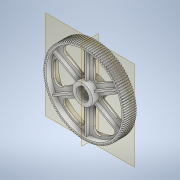
# Autodesk Inventor part: 正齿轮2
Saved by Autodesk Inventor 2020 (Build 240168000, 168)
## iProperties
CustomPartVersion: 1
Created: 2021-06-09
Part Number: 正齿轮2
Material: Steel
Document SubType Name: Modeling
Designer: dell
Categories: <?xml version="1.0" encoding="UTF-16"?> <MemberInstance><Categories><FamilyTemplate><FamilyTemplateParameter ValueType="xs:double" Id="1" ObjectReferenceKey="da_z" ObjectType="kUserParameterObject"/><FamilyTemplateParameter ValueType="xs:double" Id="2" ObjectReferenceKey="da_b" ObjectType="kUserParameterObject"/><FamilyTemplateParameter ValueType="xs:double" Id="3" ObjectReferenceKey="da_beta" ObjectType="kUserParameterObject"/><FamilyTemplateParameter ValueType="xs:double" Id="4" ObjectReferenceKey="da_da" ObjectType="kUserParameterObject"/><FamilyTemplateParameter ValueType="xs:double" Id="5" ObjectReferenceKey="da_aw" ObjectType="kUserParameterObject"/><FamilyTemplateParameter ValueType="xs:string" Id="6" ObjectReferenceKey="EAIAABAAAACIAQAAAAAAAIAAAAAAAAAA" ObjectType="83910656" SubObjectId="SurfaceGeometry"/></FamilyTemplate><ParamToTemplateMap><ParamToTemplate CategoryParameter="//CategoryParameter[@InternalName='046C89C9-8512-4d59-83FE-43B91F4F132A']" TemplateParameter="1"/><ParamToTemplate CategoryParameter="//CategoryParameter[@InternalName='2552DF32-E462-4b46-AEBF-C6C7768E72AC']" TemplateParameter="2"/><ParamToTemplate CategoryParameter="//CategoryParameter[@InternalName='C9EE641D-15FC-4fae-A226-E94C4372FDD7']" TemplateParameter="3"/><ParamToTemplate><ParamToTemplate CategoryParameter="//CategoryParameter[@InternalName='00B6519A-459B-49c7-AD84-2E56D39A5744']" ConstantValue="0.000000"/></ParamToTemplate><ParamToTemplate><ParamToTemplate CategoryParameter="//CategoryParameter[@InternalName='04B31F0E-C7A6-4894-AA32-9629BEFACF47']" ConstantValue="1.000000"/></ParamToTemplate><ParamToTemplate><ParamToTemplate CategoryParameter="//CategoryParameter[@InternalName='43CBEC2E-7847-49e7-A936-2F7889FCB2D9']" ConstantValue="0.250000"/></ParamToTemplate><ParamToTemplate><ParamToTemplate CategoryParameter="//CategoryParameter[@InternalName='B1EFC894-105D-4ebd-86BF-FA20ED196853']" ConstantValue="0.350000"/></ParamToTemplate><ParamToTemplate><ParamToTemplate CategoryParameter="//CategoryParameter[@InternalName='51175063-3D10-4879-93E8-6246FE8B403D']" ConstantValue="2060000000.000000"/></ParamToTemplate><ParamToTemplate><ParamToTemplate CategoryParameter="//CategoryParameter[@InternalName='A3A52E27-4454-46a9-B0BD-C932399B70AF']" ConstantValue="0.300000"/></ParamToTemplate><ParamToTemplate><ParamToTemplate CategoryParameter="//CategoryParameter[@InternalName='91B76062-C214-41d9-B1B9-14D2AB99603D']" ConstantValue="0.400000"/></ParamToTemplate><ParamToTemplate><ParamToTemplate CategoryParameter="//CategoryParameter[@InternalName='374E806E-8B8A-4dda-A9AA-1039D6500AD2']" ConstantValue="2.500000"/></ParamToTemplate><ParamToTemplate><ParamToTemplate CategoryParameter="//CategoryParameter[@InternalName='2D373A89-B862-43d6-8D0B-0CBF12AB9F6C']" ConstantValue="0.349066"/></ParamToTemplate><ParamToTemplate CategoryParameter="//CategoryParameter[@InternalName='37777632-D6A2-4fac-9D53-DB8ACD95C989']" TemplateParameter="4"/><ParamToTemplate CategoryParameter="//CategoryParameter[@InternalName='FD1017F1-B727-4f7e-9707-0F86F1FF9423']" TemplateParameter="5"/><ParamToTemplate><ParamToTemplate CategoryParameter="//CategoryParameter[@InternalName='9E1B4470-B2D3-4ff1-B813-535BB4CDF51A']" ConstantValue="3960000.000000"/></ParamToTemplate><ParamToTemplate><ParamToTemplate CategoryParameter="//CategoryParameter[@InternalName='F8452263-BFF6-458c-9FB1-07C4B99E95CD']" ConstantValue="4800000.000000"/></ParamToTemplate><ParamToTemplate><ParamToTemplate CategoryParameter="//CategoryParameter[@InternalName='3E3BB259-FD49-497f-8171-6EBC954A3479']" ConstantValue="0.000000"/></ParamToTemplate><ParamToTemplate CategoryParameter="//CategoryParameter[@InternalName='27C3BAF2-7550-4e4b-AE2C-0DB134B7D9B7']" TemplateParameter="6"/></ParamToTemplateMap><Category DisplayName="Gear" InternalName="DC85795E-93AB-48d5-8EEE-5A27447B64BD" Mnemonic="Gear"><CategoryParameter DisplayName="z" InternalName="046C89C9-8512-4d59-83FE-43B91F4F132A" Mnemonic="z"/><CategoryParameter DisplayName="b" InternalName="2552DF32-E462-4b46-AEBF-C6C7768E72AC" Mnemonic="b"/><CategoryParameter DisplayName="||b|" InternalName="C9EE641D-15FC-4fae-A226-E94C4372FDD7" Mnemonic="beta"/><CategoryParameter DisplayName="x" InternalName="00B6519A-459B-49c7-AD84-2E56D39A5744" Mnemonic="x"/><CategoryParameter DisplayName="a*" InternalName="04B31F0E-C7A6-4894-AA32-9629BEFACF47" Mnemonic="a"/><CategoryParameter DisplayName="c*" InternalName="43CBEC2E-7847-49e7-A936-2F7889FCB2D9" Mnemonic="c"/><CategoryParameter DisplayName="r|.f|*" InternalName="B1EFC894-105D-4ebd-86BF-FA20ED196853" Mnemonic="rf"/><CategoryParameter DisplayName="E" InternalName="51175063-3D10-4879-93E8-6246FE8B403D" Mnemonic="E"/><CategoryParameter DisplayName="||m|" InternalName="A3A52E27-4454-46a9-B0BD-C932399B70AF" Mnemonic="mi"/><Category DisplayName="SpurGear" InternalName="26C5A22E-A91E-4dfd-A3B3-23CCAFAE1764" Mnemonic="SpurGear"><CategoryParameter DisplayName="m" InternalName="91B76062-C214-41d9-B1B9-14D2AB99603D" Mnemonic="m"/><CategoryParameter DisplayName="P" InternalName="374E806E-8B8A-4dda-A9AA-1039D6500AD2" Mnemonic="PP"/><CategoryParameter DisplayName="||a|" InternalName="2D373A89-B862-43d6-8D0B-0CBF12AB9F6C" Mnemonic="alpha"/><CategoryParameter DisplayName="d|.a|" InternalName="37777632-D6A2-4fac-9D53-DB8ACD95C989" Mnemonic="da"/><CategoryParameter DisplayName="a|.w|" InternalName="FD1017F1-B727-4f7e-9707-0F86F1FF9423" Mnemonic="aw"/><CategoryParameter DisplayName="||s||.Flim|" InternalName="9E1B4470-B2D3-4ff1-B813-535BB4CDF51A" Mnemonic="sFlim"/><CategoryParameter DisplayName="||s||.Hlim|" InternalName="F8452263-BFF6-458c-9FB1-07C4B99E95CD" Mnemonic="sHlim"/><CategoryParameter DisplayName="类型" InternalName="3E3BB259-FD49-497f-8171-6EBC954A3479" Mnemonic="type"/><CategoryParameter DisplayName="PitchDiameter" InternalName="27C3BAF2-7550-4e4b-AE2C-0DB134B7D9B7" Mnemonic="IDS_PITCHDIAM"/></Category></Category></Categories></MemberInstance>
Density: 1 g/cm^3
Appearance: Steel
Author: dell
Autodesk Inventor part; units mm, degrees
(part 1 of 2)
sketch "Sketch1" plane through (0, 0, 0) normal (0, 0, 1) x (1, 0, 0)
  circle A0 centre (0, 0) radius 242
  dimension "d0" = 484
  constraints: 1 centre point
  measures "d0" diameter of A0
extrude "Extrusion1" add sketch "Sketch1" along normal blind 73
ref_plane "Work Plane2" through (0, 0, 36.5) normal (0, 0, 1) x (1, 0, 0)
sketch "Sketch2" plane through (0, 0, 0) normal (0, 0, -1) x (-1, 0, 0)
  circle A0 centre (0, 0) radius 242 projected
  circle A1 centre (0, 0) radius 238
  dimension "d3" = 476
  constraints: 1 centre point, 1 coincident
  measures "d3" diameter of A1
surface extrude "中径" sketch "Sketch2" against normal through all shown no curves A1
ref_plane "Work Plane8" through (0, 0, 0) normal (0.9996515, 0.0263969, 0) x (0, 0, 1)
ref_plane "Work Plane9" through (0, 0, 0) normal (1, 0, 0) x (0, 1, 0)
spur gear teeth "正齿轮" teeth 119 pitch diameter 476 tip diameter 484 root diameter 466 face width 73 start plane through (0, 0, 0) normal (0, 0, -1) x (-1, 0, 0)
sketch "草图3" plane through (0, 0, 73) normal (0, 0, 1) x (1, 0, 0)
  circle A0 centre (0, 0) radius 37.5
  circle A1 centre (0, 0) radius 60
  line L0 (43.1421, 10) -> (31.1421, 10)
  line L1 (31.1421, 10) -> (31.1421, -10)
  line L2 (31.1421, -10) -> (43.1421, -10)
  line L3 (43.1421, -10) -> (43.1421, 10)
  line L4 (-338.7926, 0) -> (338.7926, 0) construction
  arc A2 (-14.3663, 241.5732) -> (-16.9009, 232.3862) centre (40.0791, 221.6091) ccw projected
  arc A3 (-16.9009, 232.3862) -> (-19.9668, 232.1429) centre (0, 0) ccw projected
  arc A4 (-19.9668, 232.1429) -> (-23.9188, 240.8151) centre (-74.5336, 212.5128) ccw projected
  arc A5 (-23.9188, 240.8151) -> (-27.0954, 240.4784) centre (0, 0) ccw projected
  arc A6 (-27.0954, 240.4784) -> (-29.1416, 231.1704) centre (28.3278, 223.4155) ccw projected
  arc A7 (-29.1416, 231.1704) -> (-32.1904, 230.7656) centre (0, 0) ccw projected
  arc A8 (-32.1904, 230.7656) -> (-36.5946, 239.2171) centre (-85.6452, 208.2831) ccw projected
  arc A9 (-36.5946, 239.2171) -> (-39.749, 238.7133) centre (0, 0) ccw projected
  arc A10 (-39.749, 238.7133) -> (-41.3011, 229.3103) centre (16.4975, 224.5992) ccw projected
  arc A11 (-41.3011, 229.3103) -> (-44.3243, 228.7452) centre (0, 0) ccw projected
  arc A12 (-44.3243, 228.7452) -> (-49.1684, 236.9525) centre (-96.518, 203.4729) ccw projected
  arc A13 (-49.1684, 236.9525) -> (-52.2918, 236.2828) centre (0, 0) ccw projected
  arc A14 (-52.2918, 236.2828) -> (-53.3455, 226.8111) centre (4.6212, 225.1568) ccw projected
  arc A15 (-53.3455, 226.8111) -> (-56.3346, 226.0872) centre (0, 0) ccw projected
  arc A16 (-56.3346, 226.0872) -> (-61.6051, 234.0274) centre (-107.1219, 198.0956) ccw projected
  arc A17 (-61.6051, 234.0274) -> (-64.6888, 233.1938) centre (0, 0) ccw projected
  arc A18 (-64.6888, 233.1938) -> (-65.2412, 223.6797) centre (-7.268, 225.0869) ccw projected
  arc A19 (-65.2412, 223.6797) -> (-68.188, 222.799) centre (0, 0) ccw projected
  arc A20 (-68.188, 222.799) -> (-73.8701, 230.45) centre (-117.4271, 192.1661) ccw projected
  arc A21 (-73.8701, 230.45) -> (-76.9055, 229.4549) centre (0, 0) ccw projected
  arc A22 (-76.9055, 229.4549) -> (-76.955, 219.9248) centre (-19.1369, 224.3897) ccw projected
  arc A23 (-76.955, 219.9248) -> (-79.8512, 218.8899) centre (0, 0) ccw projected
  arc A24 (-79.8512, 218.8899) -> (-85.9292, 226.2303) centre (-127.4051, 185.701) ccw projected
  arc A25 (-85.9292, 226.2303) -> (-88.9079, 225.0764) centre (0, 0) ccw projected
  arc A26 (-88.9079, 225.0764) -> (-88.4544, 215.557) centre (-30.9525, 223.067) ccw projected
  arc A27 (-88.4544, 215.557) -> (-91.2919, 214.3707) centre (0, 0) ccw projected
  arc A28 (-91.2919, 214.3707) -> (-97.7489, 221.3801) centre (-137.028, 178.7184) ccw projected
  arc A29 (-97.7489, 221.3801) -> (-100.6625, 220.0706) centre (0, 0) ccw projected
  arc A30 (-100.6625, 220.0706) -> (-99.7072, 210.5884) centre (-42.6818, 221.1226) ccw projected
  arc A31 (-99.7072, 210.5884) -> (-102.4782, 209.254) centre (0, 0) ccw projected
  arc A32 (-102.4782, 209.254) -> (-109.2961, 215.9129) centre (-146.269, 171.2376) ccw projected
  arc A33 (-109.2961, 215.9129) -> (-112.1365, 214.4514) centre (0, 0) ccw projected
  arc A34 (-112.1365, 214.4514) -> (-110.6821, 205.0328) centre (-54.2921, 218.5619) ccw projected
  arc A35 (-110.6821, 205.0328) -> (-113.3788, 203.554) centre (0, 0) ccw projected
  arc A36 (-113.3788, 203.554) -> (-120.5386, 209.8438) centre (-155.1023, 163.2796) ccw projected
  arc A37 (-120.5386, 209.8438) -> (-123.298, 208.2345) centre (0, 0) ccw projected
  arc A38 (-123.298, 208.2345) -> (-121.3486, 198.9058) centre (-65.7511, 215.3921) ccw projected
  arc A39 (-121.3486, 198.9058) -> (-123.9635, 197.2867) centre (0, 0) ccw projected
  arc A40 (-123.9635, 197.2867) -> (-131.4452, 203.1899) centre (-163.5033, 154.8665) ccw projected
  arc A41 (-131.4452, 203.1899) -> (-134.1158, 201.4372) centre (0, 0) ccw projected
  arc A42 (-134.1158, 201.4372) -> (-131.6768, 192.2244) centre (-77.0269, 211.6218) ccw projected
  arc A43 (-131.6768, 192.2244) -> (-134.2026, 190.4696) centre (0, 0) ccw projected
  arc A44 (-134.2026, 190.4696) -> (-141.9855, 195.9697) centre (-171.4485, 146.0217) ccw projected
  arc A45 (-141.9855, 195.9697) -> (-144.5598, 194.0785) centre (0, 0) ccw projected
  arc A46 (-144.5598, 194.0785) -> (-141.638, 185.0072) centre (-88.088, 207.2618) ccw projected
  arc A47 (-141.638, 185.0072) -> (-144.0677, 183.1216) centre (0, 0) ccw projected
  arc A48 (-144.0677, 183.1216) -> (-152.13, 188.2033) centre (-178.916, 136.77) ccw projected
  arc A49 (-152.13, 188.2033) -> (-154.6009, 186.1788) centre (0, 0) ccw projected
  arc A50 (-154.6009, 186.1788) -> (-151.2044, 177.2744) centre (-98.9035, 202.3241) ccw projected
  arc A51 (-151.2044, 177.2744) -> (-153.5312, 175.2631) centre (0, 0) ccw projected
  arc A52 (-153.5312, 175.2631) -> (-161.8505, 179.9123) centre (-185.8847, 127.137) ccw projected
  arc A53 (-161.8505, 179.9123) -> (-164.2111, 177.7602) centre (0, 0) ccw projected
  arc A54 (-164.2111, 177.7602) -> (-160.3494, 169.0475) centre (-109.4434, 196.8225) ccw projected
  arc A55 (-160.3494, 169.0475) -> (-162.5668, 166.9162) centre (0, 0) ccw projected
  arc A56 (-162.5668, 166.9162) -> (-171.1198, 171.1198) centre (-192.3354, 117.1497) ccw projected
  arc A57 (-171.1198, 171.1198) -> (-173.3636, 168.8462) centre (0, 0) ccw projected
  arc A58 (-173.3636, 168.8462) -> (-169.0475, 160.3494) centre (-119.6783, 190.7723) ccw projected
  arc A59 (-169.0475, 160.3494) -> (-171.1493, 158.1041) centre (0, 0) ccw projected
  arc A60 (-171.1493, 158.1041) -> (-179.9123, 161.8505) centre (-198.2499, 106.8359) ccw projected
  arc A61 (-179.9123, 161.8505) -> (-182.033, 159.4616) centre (0, 0) ccw projected
  arc A62 (-182.033, 159.4616) -> (-177.2744, 151.2044) centre (-129.5796, 184.1904) ccw projected
  arc A63 (-177.2744, 151.2044) -> (-179.2548, 148.8513) centre (0, 0) ccw projected
  arc A64 (-179.2548, 148.8513) -> (-188.2033, 152.13) centre (-203.612, 96.2243) ccw projected
  arc A65 (-188.2033, 152.13) -> (-190.1949, 149.6325) centre (0, 0) ccw projected
  arc A66 (-190.1949, 149.6325) -> (-185.0072, 141.638) centre (-139.1197, 177.0951) ccw projected
  arc A67 (-185.0072, 141.638) -> (-186.8607, 139.1836) centre (0, 0) ccw projected
  arc A68 (-186.8607, 139.1836) -> (-195.9697, 141.9855) centre (-208.4065, 85.3445) ccw projected
  arc A69 (-195.9697, 141.9855) -> (-197.8268, 139.3864) centre (0, 0) ccw projected
  arc A70 (-197.8268, 139.3864) -> (-192.2244, 131.6768) centre (-148.2721, 169.5062) ccw projected
  arc A71 (-192.2244, 131.6768) -> (-193.9457, 129.128) centre (0, 0) ccw projected
  arc A72 (-193.9457, 129.128) -> (-203.1899, 131.4452) centre (-212.6201, 74.2269) ccw projected
  arc A73 (-203.1899, 131.4452) -> (-204.9073, 128.7518) centre (0, 0) ccw projected
  arc A74 (-204.9073, 128.7518) -> (-198.9058, 121.3486) centre (-157.0112, 161.4448) ccw projected
  arc A75 (-198.9058, 121.3486) -> (-200.4902, 118.7125) centre (0, 0) ccw projected
  arc A76 (-200.4902, 118.7125) -> (-209.8438, 120.5386) centre (-216.2412, 62.9023) ccw projected
  arc A77 (-209.8438, 120.5386) -> (-211.4166, 117.7583) centre (0, 0) ccw projected
  arc A78 (-211.4166, 117.7583) -> (-205.0328, 110.6821) centre (-165.3127, 152.9335) ccw projected
  arc A79 (-205.0328, 110.6821) -> (-206.4759, 107.9661) centre (0, 0) ccw projected
  arc A80 (-206.4759, 107.9661) -> (-215.9129, 109.2961) centre (-219.2595, 51.4024) ccw projected
  arc A81 (-215.9129, 109.2961) -> (-217.3367, 106.4366) centre (0, 0) ccw projected
  arc A82 (-217.3367, 106.4366) -> (-210.5884, 99.7072) centre (-173.1534, 143.996) ccw projected
  arc A83 (-210.5884, 99.7072) -> (-211.8861, 96.9188) centre (0, 0) ccw projected
  arc A84 (-211.8861, 96.9188) -> (-221.3801, 97.7489) centre (-221.6667, 39.7593) ccw projected
  arc A85 (-221.3801, 97.7489) -> (-222.6511, 94.8182) centre (0, 0) ccw projected
  arc A86 (-222.6511, 94.8182) -> (-215.557, 88.4544) centre (-180.5115, 134.6571) ccw projected
  arc A87 (-215.557, 88.4544) -> (-216.7058, 85.6014) centre (0, 0) ccw projected
  arc A88 (-216.7058, 85.6014) -> (-226.2303, 85.9292) centre (-223.4561, 28.0054) ccw projected
  arc A89 (-226.2303, 85.9292) -> (-227.3449, 82.9356) centre (0, 0) ccw projected
  arc A90 (-227.3449, 82.9356) -> (-219.9248, 76.955) centre (-187.3666, 124.9429) ccw projected
  arc A91 (-219.9248, 76.955) -> (-220.9214, 74.0454) centre (0, 0) ccw projected
  arc A92 (-220.9214, 74.0454) -> (-230.45, 73.8701) centre (-224.6227, 16.1734) ccw projected
  arc A93 (-230.45, 73.8701) -> (-231.405, 70.8218) centre (0, 0) ccw projected
  arc A94 (-231.405, 70.8218) -> (-223.6797, 65.2412) centre (-193.6994, 114.8804) ccw projected
  arc A95 (-223.6797, 65.2412) -> (-224.5213, 62.283) centre (0, 0) ccw projected
  arc A96 (-224.5213, 62.283) -> (-234.0274, 61.6051) centre (-225.1632, 4.2963) ccw projected
  arc A97 (-234.0274, 61.6051) -> (-234.8201, 58.5107) centre (0, 0) ccw projected
  arc A98 (-234.8201, 58.5107) -> (-226.8111, 53.3455) centre (-199.4923, 104.4978) ccw projected
  arc A99 (-226.8111, 53.3455) -> (-227.4954, 50.347) centre (0, 0) ccw projected
  arc A100 (-227.4954, 50.347) -> (-236.9525, 49.1684) centre (-225.0762, -7.5928) ccw projected
  arc A101 (-236.9525, 49.1684) -> (-237.5808, 46.0364) centre (0, 0) ccw projected
  arc A102 (-237.5808, 46.0364) -> (-229.3103, 41.3011) centre (-204.7292, 93.8239) ccw projected
  arc A103 (-229.3103, 41.3011) -> (-229.8355, 38.2707) centre (0, 0) ccw projected
  arc A104 (-229.8355, 38.2707) -> (-239.2171, 36.5946) centre (-224.3618, -19.4607) ccw projected
  arc A105 (-239.2171, 36.5946) -> (-239.6793, 33.4338) centre (0, 0) ccw projected
  arc A106 (-239.6793, 33.4338) -> (-231.1704, 29.1416) centre (-209.3954, 82.8884) ccw projected
  arc A107 (-231.1704, 29.1416) -> (-231.5349, 26.0877) centre (0, 0) ccw projected
  arc A108 (-231.5349, 26.0877) -> (-240.8151, 23.9188) centre (-223.0221, -31.2743) ccw projected
  arc A109 (-240.8151, 23.9188) -> (-241.1098, 20.7381) centre (0, 0) ccw projected
  arc A110 (-241.1098, 20.7381) -> (-232.3862, 16.9009) centre (-213.4781, 71.722) ccw projected
  arc A111 (-232.3862, 16.9009) -> (-232.5891, 13.832) centre (0, 0) ccw projected
  arc A112 (-232.5891, 13.832) -> (-241.7418, 11.1764) centre (-221.0608, -43.0008) ccw projected
  arc A113 (-241.7418, 11.1764) -> (-241.8682, 7.9845) centre (0, 0) ccw projected
  arc A114 (-241.8682, 7.9845) -> (-232.9543, 4.6131) centre (-216.9658, 60.3557) ccw projected
  arc A115 (-232.9543, 4.6131) -> (-232.9949, 1.5378) centre (0, 0) ccw projected
  arc A116 (-232.9949, 1.5378) -> (-241.9947, -1.5972) centre (-218.4833, -54.6074) ccw projected
  arc A117 (-241.9947, -1.5972) -> (-241.9526, -4.7913) centre (0, 0) ccw projected
  arc A118 (-241.9526, -4.7913) -> (-232.8731, -7.6876) centre (-219.8487, 48.8211) ccw projected
  arc A119 (-232.8731, -7.6876) -> (-232.7514, -10.7607) centre (0, 0) ccw projected
  arc A120 (-232.7514, -10.7607) -> (-241.5732, -14.3663) centre (-215.2969, -66.0619) ccw projected
  arc A121 (-241.5732, -14.3663) -> (-241.3625, -17.5537) centre (0, 0) ccw projected
  arc A122 (-241.3625, -17.5537) -> (-232.1429, -19.9668) centre (-222.1189, 37.1505) ccw projected
  arc A123 (-232.1429, -19.9668) -> (-231.8591, -23.0293) centre (0, 0) ccw projected
  arc A124 (-231.8591, -23.0293) -> (-240.4784, -27.0954) centre (-211.5105, -77.3322) ccw projected
  arc A125 (-240.4784, -27.0954) -> (-240.0998, -30.2673) centre (0, 0) ccw projected
  arc A126 (-240.0998, -30.2673) -> (-230.7656, -32.1904) centre (-223.7699, 25.3763) ccw projected
  arc A127 (-230.7656, -32.1904) -> (-230.3206, -35.2336) centre (0, 0) ccw projected
  arc A128 (-230.3206, -35.2336) -> (-238.7133, -39.749) centre (-207.1345, -88.387) ccw projected
  arc A129 (-238.7133, -39.749) -> (-238.1678, -42.8964) centre (0, 0) ccw projected
  arc A130 (-238.1678, -42.8964) -> (-228.7452, -44.3243) centre (-224.7973, 13.5314) ccw projected
  arc A131 (-228.7452, -44.3243) -> (-228.1402, -47.3398) centre (0, 0) ccw projected
  arc A132 (-228.1402, -47.3398) -> (-236.2828, -52.2918) centre (-202.1812, -99.1954) ccw projected
  arc A133 (-236.2828, -52.2918) -> (-235.572, -55.406) centre (0, 0) ccw projected
  arc A134 (-235.572, -55.406) -> (-226.0872, -56.3346) centre (-225.1982, 1.6488) ccw projected
  arc A135 (-226.0872, -56.3346) -> (-225.3239, -59.314) centre (0, 0) ccw projected
  arc A136 (-225.3239, -59.314) -> (-233.1938, -64.6888) centre (-196.6643, -109.7273) ccw projected
  arc A137 (-233.1938, -64.6888) -> (-232.3196, -67.7612) centre (0, 0) ccw projected
  arc A138 (-232.3196, -67.7612) -> (-222.799, -68.188) centre (-224.9714, -10.2384) ccw projected
  arc A139 (-222.799, -68.188) -> (-221.8796, -71.1229) centre (0, 0) ccw projected
  arc A140 (-221.8796, -71.1229) -> (-229.4549, -76.9055) centre (-190.5994, -119.9534) ccw projected
  arc A141 (-229.4549, -76.9055) -> (-228.4198, -79.9275) centre (0, 0) ccw projected
  arc A142 (-228.4198, -79.9275) -> (-218.8899, -79.8512) centre (-224.1175, -22.0971) ccw projected
  arc A143 (-218.8899, -79.8512) -> (-217.8168, -82.7335) centre (0, 0) ccw projected
  arc A144 (-217.8168, -82.7335) -> (-225.0764, -88.9079) centre (-184.0032, -129.8452) ccw projected
  arc A145 (-225.0764, -88.9079) -> (-223.8832, -91.8711) centre (0, 0) ccw projected
  arc A146 (-223.8832, -91.8711) -> (-214.3707, -91.2919) centre (-222.639, -33.8942) ccw projected
  arc A147 (-214.3707, -91.2919) -> (-213.147, -94.1136) centre (0, 0) ccw projected
  arc A148 (-213.147, -94.1136) -> (-220.0706, -100.6625) centre (-176.8941, -139.3751) ccw projected
  arc A149 (-220.0706, -100.6625) -> (-218.7227, -103.5586) centre (0, 0) ccw projected
  arc A150 (-218.7227, -103.5586) -> (-209.254, -102.4782) centre (-220.54, -45.5968) ccw projected
  arc A151 (-209.254, -102.4782) -> (-207.8831, -105.2313) centre (0, 0) ccw projected
  arc A152 (-207.8831, -105.2313) -> (-214.4514, -112.1365) centre (-169.292, -148.5165) ccw projected
  arc A153 (-214.4514, -112.1365) -> (-212.9526, -114.9574) centre (0, 0) ccw projected
  arc A154 (-212.9526, -114.9574) -> (-203.554, -113.3788) centre (-217.8262, -57.1723) ccw projected
  arc A155 (-203.554, -113.3788) -> (-202.0397, -116.0558) centre (0, 0) ccw projected
  arc A156 (-202.0397, -116.0558) -> (-208.2345, -123.298) centre (-161.2181, -157.244) ccw projected
  arc A157 (-208.2345, -123.298) -> (-206.5889, -126.0359) centre (0, 0) ccw projected
  arc A158 (-206.5889, -126.0359) -> (-197.2867, -123.9635) centre (-214.5054, -68.5885) ccw projected
  arc A159 (-197.2867, -123.9635) -> (-195.6333, -126.5568) centre (0, 0) ccw projected
  arc A160 (-195.6333, -126.5568) -> (-201.4372, -134.1158) centre (-152.6948, -165.5332) ccw projected
  arc A161 (-201.4372, -134.1158) -> (-199.6494, -136.763) centre (0, 0) ccw projected
  arc A162 (-199.6494, -136.763) -> (-190.4696, -134.2026) centre (-210.5867, -79.8135) ccw projected
  arc A163 (-190.4696, -134.2026) -> (-188.6816, -136.705) centre (0, 0) ccw projected
  arc A164 (-188.6816, -136.705) -> (-194.0785, -144.5598) centre (-143.746, -173.361) ccw projected
  arc A165 (-194.0785, -144.5598) -> (-192.1534, -147.109) centre (0, 0) ccw projected
  arc A166 (-192.1534, -147.109) -> (-183.1216, -144.0677) centre (-206.081, -90.8161) ccw projected
  arc A167 (-183.1216, -144.0677) -> (-181.204, -146.4722) centre (0, 0) ccw projected
  arc A168 (-181.204, -146.4722) -> (-186.1788, -154.6009) centre (-134.3964, -180.7057) ccw projected
  arc A169 (-186.1788, -154.6009) -> (-184.1219, -157.0449) centre (0, 0) ccw projected
  arc A170 (-184.1219, -157.0449) -> (-175.2631, -153.5312) centre (-201.001, -101.5655) ccw projected
  arc A171 (-175.2631, -153.5312) -> (-173.2213, -155.8312) centre (0, 0) ccw projected
  arc A172 (-173.2213, -155.8312) -> (-177.7602, -164.2111) centre (-124.6724, -187.5467) ccw projected
  arc A173 (-177.7602, -164.2111) -> (-175.5772, -166.5432) centre (0, 0) ccw projected
  arc A174 (-175.5772, -166.5432) -> (-166.9162, -162.5668) centre (-195.3607, -112.0318) ccw projected
  arc A175 (-166.9162, -162.5668) -> (-164.7559, -164.7559) centre (0, 0) ccw projected
  arc A176 (-164.7559, -164.7559) -> (-168.8462, -173.3636) centre (-114.6008, -193.8649) ccw projected
  arc A177 (-168.8462, -173.3636) -> (-166.5432, -175.5772) centre (0, 0) ccw projected
  arc A178 (-166.5432, -175.5772) -> (-158.1041, -171.1493) centre (-189.1759, -122.186) ccw projected
  arc A179 (-158.1041, -171.1493) -> (-155.8312, -173.2213) centre (0, 0) ccw projected
  arc A180 (-155.8312, -173.2213) -> (-159.4616, -182.033) centre (-104.2098, -199.6429) ccw projected
  arc A181 (-159.4616, -182.033) -> (-157.0449, -184.1219) centre (0, 0) ccw projected
  arc A182 (-157.0449, -184.1219) -> (-148.8513, -179.2548) centre (-182.4639, -131.9995) ccw projected
  arc A183 (-148.8513, -179.2548) -> (-146.4722, -181.204) centre (0, 0) ccw projected
  arc A184 (-146.4722, -181.204) -> (-149.6325, -190.1949) centre (-93.5283, -204.8643) ccw projected
  arc A185 (-149.6325, -190.1949) -> (-147.109, -192.1534) centre (0, 0) ccw projected
  arc A186 (-147.109, -192.1534) -> (-139.1836, -186.8607) centre (-175.2433, -141.4451) ccw projected
  arc A187 (-139.1836, -186.8607) -> (-136.705, -188.6816) centre (0, 0) ccw projected
  arc A188 (-136.705, -188.6816) -> (-139.3864, -197.8268) centre (-82.5862, -209.5148) ccw projected
  arc A189 (-139.3864, -197.8268) -> (-136.763, -199.6494) centre (0, 0) ccw projected
  arc A190 (-136.763, -199.6494) -> (-129.128, -193.9457) centre (-167.5343, -150.4966) ccw projected
  arc A191 (-129.128, -193.9457) -> (-126.5568, -195.6333) centre (0, 0) ccw projected
  arc A192 (-126.5568, -195.6333) -> (-128.7518, -204.9073) centre (-71.4139, -213.5814) ccw projected
  arc A193 (-128.7518, -204.9073) -> (-126.0359, -206.5889) centre (0, 0) ccw projected
  arc A194 (-126.0359, -206.5889) -> (-118.7125, -200.4902) centre (-159.3583, -159.1285) ccw projected
  arc A195 (-118.7125, -200.4902) -> (-116.0558, -202.0397) centre (0, 0) ccw projected
  arc A196 (-116.0558, -202.0397) -> (-117.7583, -211.4166) centre (-60.0425, -217.0526) ccw projected
  arc A197 (-117.7583, -211.4166) -> (-114.9574, -212.9526) centre (0, 0) ccw projected
  arc A198 (-114.9574, -212.9526) -> (-107.9661, -206.4759) centre (-150.7382, -167.3169) ccw projected
  arc A199 (-107.9661, -206.4759) -> (-105.2313, -207.8831) centre (0, 0) ccw projected
  arc A200 (-105.2313, -207.8831) -> (-106.4366, -217.3367) centre (-48.5038, -219.9189) ccw projected
  arc A201 (-106.4366, -217.3367) -> (-103.5586, -218.7227) centre (0, 0) ccw projected
  arc A202 (-103.5586, -218.7227) -> (-96.9188, -211.8861) centre (-141.6979, -175.039) ccw projected
  arc A203 (-96.9188, -211.8861) -> (-94.1136, -213.147) centre (0, 0) ccw projected
  arc A204 (-94.1136, -213.147) -> (-94.8182, -222.6511) centre (-36.8299, -222.1722) ccw projected
  arc A205 (-94.8182, -222.6511) -> (-91.8711, -223.8832) centre (0, 0) ccw projected
  arc A206 (-91.8711, -223.8832) -> (-85.6014, -216.7058) centre (-132.2627, -182.2732) ccw projected
  arc A207 (-85.6014, -216.7058) -> (-82.7335, -217.8168) centre (0, 0) ccw projected
  arc A208 (-82.7335, -217.8168) -> (-82.9356, -227.3449) centre (-25.0534, -223.8063) ccw projected
  arc A209 (-82.9356, -227.3449) -> (-79.9275, -228.4198) centre (0, 0) ccw projected
  arc A210 (-79.9275, -228.4198) -> (-74.0454, -220.9214) centre (-122.4588, -188.9994) ccw projected
  arc A211 (-74.0454, -220.9214) -> (-71.1229, -221.8796) centre (0, 0) ccw projected
  arc A212 (-71.1229, -221.8796) -> (-70.8218, -231.405) centre (-13.207, -224.8166) ccw projected
  arc A213 (-70.8218, -231.405) -> (-67.7612, -232.3196) centre (0, 0) ccw projected
  arc A214 (-67.7612, -232.3196) -> (-62.283, -224.5213) centre (-112.3136, -195.1989) ccw projected
  arc A215 (-62.283, -224.5213) -> (-59.314, -225.3239) centre (0, 0) ccw projected
  arc A216 (-59.314, -225.3239) -> (-58.5107, -234.8201) centre (-1.3238, -225.2003) ccw projected
  arc A217 (-58.5107, -234.8201) -> (-55.406, -235.572) centre (0, 0) ccw projected
  arc A218 (-55.406, -235.572) -> (-50.347, -227.4954) centre (-101.8554, -200.8542) ccw projected
  arc A219 (-50.347, -227.4954) -> (-47.3398, -228.1402) centre (0, 0) ccw projected
  arc A220 (-47.3398, -228.1402) -> (-46.0364, -237.5808) centre (10.563, -224.9564) ccw projected
  arc A221 (-46.0364, -237.5808) -> (-42.8964, -238.1678) centre (0, 0) ccw projected
  arc A222 (-42.8964, -238.1678) -> (-38.2707, -229.8355) centre (-91.1133, -205.9498) ccw projected
  arc A223 (-38.2707, -229.8355) -> (-35.2336, -230.3206) centre (0, 0) ccw projected
  arc A224 (-35.2336, -230.3206) -> (-33.4338, -239.6793) centre (22.4205, -224.0854) ccw projected
  arc A225 (-33.4338, -239.6793) -> (-30.2673, -240.0998) centre (0, 0) ccw projected
  arc A226 (-30.2673, -240.0998) -> (-26.0877, -231.5349) centre (-80.1173, -210.4713) ccw projected
  arc A227 (-26.0877, -231.5349) -> (-23.0293, -231.8591) centre (0, 0) ccw projected
  arc A228 (-23.0293, -231.8591) -> (-20.7381, -241.1098) centre (34.2154, -222.5899) ccw projected
  arc A229 (-20.7381, -241.1098) -> (-17.5537, -241.3625) centre (0, 0) ccw projected
  arc A230 (-17.5537, -241.3625) -> (-13.832, -232.5891) centre (-68.8979, -214.4062) ccw projected
  arc A231 (-13.832, -232.5891) -> (-10.7607, -232.7514) centre (0, 0) ccw projected
  arc A232 (-10.7607, -232.7514) -> (-7.9845, -241.8682) centre (45.915, -220.4739) ccw projected
  arc A233 (-7.9845, -241.8682) -> (-4.7913, -241.9526) centre (0, 0) ccw projected
  arc A234 (-4.7913, -241.9526) -> (-1.5378, -232.9949) centre (-57.4866, -217.7435) ccw projected
  arc A235 (-1.5378, -232.9949) -> (1.5378, -232.9949) centre (0, 0) ccw projected
  arc A236 (1.5378, -232.9949) -> (4.7913, -241.9526) centre (57.4866, -217.7435) ccw projected
  arc A237 (4.7913, -241.9526) -> (7.9845, -241.8682) centre (0, 0) ccw projected
  arc A238 (7.9845, -241.8682) -> (10.7607, -232.7514) centre (-45.915, -220.4739) ccw projected
  arc A239 (10.7607, -232.7514) -> (13.832, -232.5891) centre (0, 0) ccw projected
  arc A240 (13.832, -232.5891) -> (17.5537, -241.3625) centre (68.8979, -214.4062) ccw projected
  arc A241 (17.5537, -241.3625) -> (20.7381, -241.1098) centre (0, 0) ccw projected
  arc A242 (20.7381, -241.1098) -> (23.0293, -231.8591) centre (-34.2154, -222.5899) ccw projected
  arc A243 (23.0293, -231.8591) -> (26.0877, -231.5349) centre (0, 0) ccw projected
  arc A244 (26.0877, -231.5349) -> (30.2673, -240.0998) centre (80.1173, -210.4713) ccw projected
  arc A245 (30.2673, -240.0998) -> (33.4338, -239.6793) centre (0, 0) ccw projected
  arc A246 (33.4338, -239.6793) -> (35.2336, -230.3206) centre (-22.4205, -224.0854) ccw projected
  arc A247 (35.2336, -230.3206) -> (38.2707, -229.8355) centre (0, 0) ccw projected
  arc A248 (38.2707, -229.8355) -> (42.8964, -238.1678) centre (91.1133, -205.9498) ccw projected
  arc A249 (42.8964, -238.1678) -> (46.0364, -237.5808) centre (0, 0) ccw projected
  arc A250 (46.0364, -237.5808) -> (47.3398, -228.1402) centre (-10.563, -224.9564) ccw projected
  arc A251 (47.3398, -228.1402) -> (50.347, -227.4954) centre (0, 0) ccw projected
  arc A252 (50.347, -227.4954) -> (55.406, -235.572) centre (101.8554, -200.8542) ccw projected
  arc A253 (55.406, -235.572) -> (58.5107, -234.8201) centre (0, 0) ccw projected
  arc A254 (58.5107, -234.8201) -> (59.314, -225.3239) centre (1.3238, -225.2003) ccw projected
  arc A255 (59.314, -225.3239) -> (62.283, -224.5213) centre (0, 0) ccw projected
  arc A256 (62.283, -224.5213) -> (67.7612, -232.3196) centre (112.3136, -195.1989) ccw projected
  arc A257 (67.7612, -232.3196) -> (70.8218, -231.405) centre (0, 0) ccw projected
  arc A258 (70.8218, -231.405) -> (71.1229, -221.8796) centre (13.207, -224.8166) ccw projected
  arc A259 (71.1229, -221.8796) -> (74.0454, -220.9214) centre (0, 0) ccw projected
  arc A260 (74.0454, -220.9214) -> (79.9275, -228.4198) centre (122.4588, -188.9994) ccw projected
  arc A261 (79.9275, -228.4198) -> (82.9356, -227.3449) centre (0, 0) ccw projected
  arc A262 (82.9356, -227.3449) -> (82.7335, -217.8168) centre (25.0534, -223.8063) ccw projected
  arc A263 (82.7335, -217.8168) -> (85.6014, -216.7058) centre (0, 0) ccw projected
  arc A264 (85.6014, -216.7058) -> (91.8711, -223.8832) centre (132.2627, -182.2732) ccw projected
  arc A265 (91.8711, -223.8832) -> (94.8182, -222.6511) centre (0, 0) ccw projected
  arc A266 (94.8182, -222.6511) -> (94.1136, -213.147) centre (36.8299, -222.1722) ccw projected
  arc A267 (94.1136, -213.147) -> (96.9188, -211.8861) centre (0, 0) ccw projected
  arc A268 (96.9188, -211.8861) -> (103.5586, -218.7227) centre (141.6979, -175.039) ccw projected
  arc A269 (103.5586, -218.7227) -> (106.4366, -217.3367) centre (0, 0) ccw projected
  arc A270 (106.4366, -217.3367) -> (105.2313, -207.8831) centre (48.5038, -219.9189) ccw projected
  arc A271 (105.2313, -207.8831) -> (107.9661, -206.4759) centre (0, 0) ccw projected
  arc A272 (107.9661, -206.4759) -> (114.9574, -212.9526) centre (150.7382, -167.3169) ccw projected
  arc A273 (114.9574, -212.9526) -> (117.7583, -211.4166) centre (0, 0) ccw projected
  arc A274 (117.7583, -211.4166) -> (116.0558, -202.0397) centre (60.0425, -217.0526) ccw projected
  arc A275 (116.0558, -202.0397) -> (118.7125, -200.4902) centre (0, 0) ccw projected
  arc A276 (118.7125, -200.4902) -> (126.0359, -206.5889) centre (159.3583, -159.1285) ccw projected
  arc A277 (126.0359, -206.5889) -> (128.7518, -204.9073) centre (0, 0) ccw projected
  arc A278 (128.7518, -204.9073) -> (126.5568, -195.6333) centre (71.4139, -213.5814) ccw projected
  arc A279 (126.5568, -195.6333) -> (129.128, -193.9457) centre (0, 0) ccw projected
  arc A280 (129.128, -193.9457) -> (136.763, -199.6494) centre (167.5343, -150.4966) ccw projected
  arc A281 (136.763, -199.6494) -> (139.3864, -197.8268) centre (0, 0) ccw projected
  arc A282 (139.3864, -197.8268) -> (136.705, -188.6816) centre (82.5862, -209.5148) ccw projected
  arc A283 (136.705, -188.6816) -> (139.1836, -186.8607) centre (0, 0) ccw projected
  arc A284 (139.1836, -186.8607) -> (147.109, -192.1534) centre (175.2433, -141.4451) ccw projected
  arc A285 (147.109, -192.1534) -> (149.6325, -190.1949) centre (0, 0) ccw projected
  arc A286 (149.6325, -190.1949) -> (146.4722, -181.204) centre (93.5283, -204.8643) ccw projected
  arc A287 (146.4722, -181.204) -> (148.8513, -179.2548) centre (0, 0) ccw projected
  arc A288 (148.8513, -179.2548) -> (157.0449, -184.1219) centre (182.4639, -131.9995) ccw projected
  arc A289 (157.0449, -184.1219) -> (159.4616, -182.033) centre (0, 0) ccw projected
  arc A290 (159.4616, -182.033) -> (155.8312, -173.2213) centre (104.2098, -199.6429) ccw projected
  arc A291 (155.8312, -173.2213) -> (158.1041, -171.1493) centre (0, 0) ccw projected
  arc A292 (158.1041, -171.1493) -> (166.5432, -175.5772) centre (189.1759, -122.186) ccw projected
  arc A293 (166.5432, -175.5772) -> (168.8462, -173.3636) centre (0, 0) ccw projected
  arc A294 (168.8462, -173.3636) -> (164.7559, -164.7559) centre (114.6008, -193.8649) ccw projected
  arc A295 (164.7559, -164.7559) -> (166.9162, -162.5668) centre (0, 0) ccw projected
  arc A296 (166.9162, -162.5668) -> (175.5772, -166.5432) centre (195.3607, -112.0318) ccw projected
  arc A297 (175.5772, -166.5432) -> (177.7602, -164.2111) centre (0, 0) ccw projected
  arc A298 (177.7602, -164.2111) -> (173.2213, -155.8312) centre (124.6724, -187.5467) ccw projected
  arc A299 (173.2213, -155.8312) -> (175.2631, -153.5312) centre (0, 0) ccw projected
  arc A300 (175.2631, -153.5312) -> (184.1219, -157.0449) centre (201.001, -101.5655) ccw projected
  arc A301 (184.1219, -157.0449) -> (186.1788, -154.6009) centre (0, 0) ccw projected
  arc A302 (186.1788, -154.6009) -> (181.204, -146.4722) centre (134.3964, -180.7057) ccw projected
  arc A303 (181.204, -146.4722) -> (183.1216, -144.0677) centre (0, 0) ccw projected
  arc A304 (183.1216, -144.0677) -> (192.1534, -147.109) centre (206.081, -90.8161) ccw projected
  arc A305 (192.1534, -147.109) -> (194.0785, -144.5598) centre (0, 0) ccw projected
  arc A306 (194.0785, -144.5598) -> (188.6816, -136.705) centre (143.746, -173.361) ccw projected
  arc A307 (188.6816, -136.705) -> (190.4696, -134.2026) centre (0, 0) ccw projected
  arc A308 (190.4696, -134.2026) -> (199.6494, -136.763) centre (210.5867, -79.8135) ccw projected
  arc A309 (199.6494, -136.763) -> (201.4372, -134.1158) centre (0, 0) ccw projected
  arc A310 (201.4372, -134.1158) -> (195.6333, -126.5568) centre (152.6948, -165.5332) ccw projected
  arc A311 (195.6333, -126.5568) -> (197.2867, -123.9635) centre (0, 0) ccw projected
  arc A312 (197.2867, -123.9635) -> (206.5889, -126.0359) centre (214.5054, -68.5885) ccw projected
  arc A313 (206.5889, -126.0359) -> (208.2345, -123.298) centre (0, 0) ccw projected
  arc A314 (208.2345, -123.298) -> (202.0397, -116.0558) centre (161.2181, -157.244) ccw projected
  arc A315 (202.0397, -116.0558) -> (203.554, -113.3788) centre (0, 0) ccw projected
  arc A316 (203.554, -113.3788) -> (212.9526, -114.9574) centre (217.8262, -57.1723) ccw projected
  arc A317 (212.9526, -114.9574) -> (214.4514, -112.1365) centre (0, 0) ccw projected
  arc A318 (214.4514, -112.1365) -> (207.8831, -105.2313) centre (169.292, -148.5165) ccw projected
  arc A319 (207.8831, -105.2313) -> (209.254, -102.4782) centre (0, 0) ccw projected
  arc A320 (209.254, -102.4782) -> (218.7227, -103.5586) centre (220.54, -45.5968) ccw projected
  arc A321 (218.7227, -103.5586) -> (220.0706, -100.6625) centre (0, 0) ccw projected
  arc A322 (220.0706, -100.6625) -> (213.147, -94.1136) centre (176.8941, -139.3751) ccw projected
  arc A323 (213.147, -94.1136) -> (214.3707, -91.2919) centre (0, 0) ccw projected
  arc A324 (214.3707, -91.2919) -> (223.8832, -91.8711) centre (222.639, -33.8942) ccw projected
  arc A325 (223.8832, -91.8711) -> (225.0764, -88.9079) centre (0, 0) ccw projected
  arc A326 (225.0764, -88.9079) -> (217.8168, -82.7335) centre (184.0032, -129.8452) ccw projected
  arc A327 (217.8168, -82.7335) -> (218.8899, -79.8512) centre (0, 0) ccw projected
  arc A328 (218.8899, -79.8512) -> (228.4198, -79.9275) centre (224.1175, -22.0971) ccw projected
  arc A329 (228.4198, -79.9275) -> (229.4549, -76.9055) centre (0, 0) ccw projected
  arc A330 (229.4549, -76.9055) -> (221.8796, -71.1229) centre (190.5994, -119.9534) ccw projected
  arc A331 (221.8796, -71.1229) -> (222.799, -68.188) centre (0, 0) ccw projected
  arc A332 (222.799, -68.188) -> (232.3196, -67.7612) centre (224.9714, -10.2384) ccw projected
  arc A333 (232.3196, -67.7612) -> (233.1938, -64.6888) centre (0, 0) ccw projected
  arc A334 (233.1938, -64.6888) -> (225.3239, -59.314) centre (196.6643, -109.7273) ccw projected
  arc A335 (225.3239, -59.314) -> (226.0872, -56.3346) centre (0, 0) ccw projected
  arc A336 (226.0872, -56.3346) -> (235.572, -55.406) centre (225.1982, 1.6488) ccw projected
  arc A337 (235.572, -55.406) -> (236.2828, -52.2918) centre (0, 0) ccw projected
  arc A338 (236.2828, -52.2918) -> (228.1402, -47.3398) centre (202.1812, -99.1954) ccw projected
  arc A339 (228.1402, -47.3398) -> (228.7452, -44.3243) centre (0, 0) ccw projected
  arc A340 (228.7452, -44.3243) -> (238.1678, -42.8964) centre (224.7973, 13.5314) ccw projected
  arc A341 (238.1678, -42.8964) -> (238.7133, -39.749) centre (0, 0) ccw projected
  arc A342 (238.7133, -39.749) -> (230.3206, -35.2336) centre (207.1345, -88.387) ccw projected
  arc A343 (230.3206, -35.2336) -> (230.7656, -32.1904) centre (0, 0) ccw projected
  arc A344 (230.7656, -32.1904) -> (240.0998, -30.2673) centre (223.7699, 25.3763) ccw projected
  arc A345 (240.0998, -30.2673) -> (240.4784, -27.0954) centre (0, 0) ccw projected
  arc A346 (240.4784, -27.0954) -> (231.8591, -23.0293) centre (211.5105, -77.3322) ccw projected
  arc A347 (231.8591, -23.0293) -> (232.1429, -19.9668) centre (0, 0) ccw projected
  arc A348 (232.1429, -19.9668) -> (241.3625, -17.5537) centre (222.1189, 37.1505) ccw projected
  arc A349 (241.3625, -17.5537) -> (241.5732, -14.3663) centre (0, 0) ccw projected
  arc A350 (241.5732, -14.3663) -> (232.7514, -10.7607) centre (215.2969, -66.0619) ccw projected
  arc A351 (232.7514, -10.7607) -> (232.8731, -7.6876) centre (0, 0) ccw projected
  arc A352 (232.8731, -7.6876) -> (241.9526, -4.7913) centre (219.8487, 48.8211) ccw projected
  arc A353 (241.9526, -4.7913) -> (241.9947, -1.5972) centre (0, 0) ccw projected
  arc A354 (241.9947, -1.5972) -> (232.9949, 1.5378) centre (218.4833, -54.6074) ccw projected
  arc A355 (232.9949, 1.5378) -> (232.9543, 4.6131) centre (0, 0) ccw projected
  arc A356 (232.9543, 4.6131) -> (241.8682, 7.9845) centre (216.9658, 60.3557) ccw projected
  arc A357 (241.8682, 7.9845) -> (241.7418, 11.1764) centre (0, 0) ccw projected
  arc A358 (241.7418, 11.1764) -> (232.5891, 13.832) centre (221.0608, -43.0008) ccw projected
  arc A359 (232.5891, 13.832) -> (232.3862, 16.9009) centre (0, 0) ccw projected
  arc A360 (232.3862, 16.9009) -> (241.1098, 20.7381) centre (213.4781, 71.722) ccw projected
  arc A361 (241.1098, 20.7381) -> (240.8151, 23.9188) centre (0, 0) ccw projected
  arc A362 (240.8151, 23.9188) -> (231.5349, 26.0877) centre (223.0221, -31.2743) ccw projected
  arc A363 (231.5349, 26.0877) -> (231.1704, 29.1416) centre (0, 0) ccw projected
  arc A364 (231.1704, 29.1416) -> (239.6793, 33.4338) centre (209.3954, 82.8884) ccw projected
  arc A365 (239.6793, 33.4338) -> (239.2171, 36.5946) centre (0, 0) ccw projected
  arc A366 (239.2171, 36.5946) -> (229.8355, 38.2707) centre (224.3618, -19.4607) ccw projected
  arc A367 (229.8355, 38.2707) -> (229.3103, 41.3011) centre (0, 0) ccw projected
  arc A368 (229.3103, 41.3011) -> (237.5808, 46.0364) centre (204.7292, 93.8239) ccw projected
  arc A369 (237.5808, 46.0364) -> (236.9525, 49.1684) centre (0, 0) ccw projected
  arc A370 (236.9525, 49.1684) -> (227.4954, 50.347) centre (225.0762, -7.5928) ccw projected
  arc A371 (227.4954, 50.347) -> (226.8111, 53.3455) centre (0, 0) ccw projected
  arc A372 (226.8111, 53.3455) -> (234.8201, 58.5107) centre (199.4923, 104.4978) ccw projected
  arc A373 (234.8201, 58.5107) -> (234.0274, 61.6051) centre (0, 0) ccw projected
  arc A374 (234.0274, 61.6051) -> (224.5213, 62.283) centre (225.1632, 4.2963) ccw projected
  arc A375 (224.5213, 62.283) -> (223.6797, 65.2412) centre (0, 0) ccw projected
  arc A376 (223.6797, 65.2412) -> (231.405, 70.8218) centre (193.6994, 114.8804) ccw projected
  arc A377 (231.405, 70.8218) -> (230.45, 73.8701) centre (0, 0) ccw projected
  arc A378 (230.45, 73.8701) -> (220.9214, 74.0454) centre (224.6227, 16.1734) ccw projected
  arc A379 (220.9214, 74.0454) -> (219.9248, 76.955) centre (0, 0) ccw projected
  arc A380 (219.9248, 76.955) -> (227.3449, 82.9356) centre (187.3666, 124.9429) ccw projected
  arc A381 (227.3449, 82.9356) -> (226.2303, 85.9292) centre (0, 0) ccw projected
  arc A382 (226.2303, 85.9292) -> (216.7058, 85.6014) centre (223.4561, 28.0054) ccw projected
  arc A383 (216.7058, 85.6014) -> (215.557, 88.4544) centre (0, 0) ccw projected
  arc A384 (215.557, 88.4544) -> (222.6511, 94.8182) centre (180.5115, 134.6571) ccw projected
  arc A385 (222.6511, 94.8182) -> (221.3801, 97.7489) centre (0, 0) ccw projected
  arc A386 (221.3801, 97.7489) -> (211.8861, 96.9188) centre (221.6667, 39.7593) ccw projected
  arc A387 (211.8861, 96.9188) -> (210.5884, 99.7072) centre (0, 0) ccw projected
  arc A388 (210.5884, 99.7072) -> (217.3367, 106.4366) centre (173.1534, 143.996) ccw projected
  arc A389 (217.3367, 106.4366) -> (215.9129, 109.2961) centre (0, 0) ccw projected
  arc A390 (215.9129, 109.2961) -> (206.4759, 107.9661) centre (219.2595, 51.4024) ccw projected
  arc A391 (206.4759, 107.9661) -> (205.0328, 110.6821) centre (0, 0) ccw projected
  arc A392 (205.0328, 110.6821) -> (211.4166, 117.7583) centre (165.3127, 152.9335) ccw projected
  arc A393 (211.4166, 117.7583) -> (209.8438, 120.5386) centre (0, 0) ccw projected
  arc A394 (209.8438, 120.5386) -> (200.4902, 118.7125) centre (216.2412, 62.9023) ccw projected
  arc A395 (200.4902, 118.7125) -> (198.9058, 121.3486) centre (0, 0) ccw projected
  arc A396 (198.9058, 121.3486) -> (204.9073, 128.7518) centre (157.0112, 161.4448) ccw projected
  arc A397 (204.9073, 128.7518) -> (203.1899, 131.4452) centre (0, 0) ccw projected
  arc A398 (203.1899, 131.4452) -> (193.9457, 129.128) centre (212.6201, 74.2269) ccw projected
  arc A399 (193.9457, 129.128) -> (192.2244, 131.6768) centre (0, 0) ccw projected
  arc A400 (192.2244, 131.6768) -> (197.8268, 139.3864) centre (148.2721, 169.5062) ccw projected
  arc A401 (197.8268, 139.3864) -> (195.9697, 141.9855) centre (0, 0) ccw projected
  arc A402 (195.9697, 141.9855) -> (186.8607, 139.1836) centre (208.4065, 85.3445) ccw projected
  arc A403 (186.8607, 139.1836) -> (185.0072, 141.638) centre (0, 0) ccw projected
  arc A404 (185.0072, 141.638) -> (190.1949, 149.6325) centre (139.1197, 177.0951) ccw projected
  arc A405 (190.1949, 149.6325) -> (188.2033, 152.13) centre (0, 0) ccw projected
  arc A406 (188.2033, 152.13) -> (179.2548, 148.8513) centre (203.612, 96.2243) ccw projected
  arc A407 (179.2548, 148.8513) -> (177.2744, 151.2044) centre (0, 0) ccw projected
  arc A408 (177.2744, 151.2044) -> (182.033, 159.4616) centre (129.5796, 184.1904) ccw projected
  arc A409 (182.033, 159.4616) -> (179.9123, 161.8505) centre (0, 0) ccw projected
  arc A410 (179.9123, 161.8505) -> (171.1493, 158.1041) centre (198.2499, 106.8359) ccw projected
  arc A411 (171.1493, 158.1041) -> (169.0475, 160.3494) centre (0, 0) ccw projected
  arc A412 (169.0475, 160.3494) -> (173.3636, 168.8462) centre (119.6783, 190.7723) ccw projected
  arc A413 (173.3636, 168.8462) -> (171.1198, 171.1198) centre (0, 0) ccw projected
  arc A414 (171.1198, 171.1198) -> (162.5668, 166.9162) centre (192.3354, 117.1497) ccw projected
  arc A415 (162.5668, 166.9162) -> (160.3494, 169.0475) centre (0, 0) ccw projected
  arc A416 (160.3494, 169.0475) -> (164.2111, 177.7602) centre (109.4434, 196.8225) ccw projected
  arc A417 (164.2111, 177.7602) -> (161.8505, 179.9123) centre (0, 0) ccw projected
  arc A418 (161.8505, 179.9123) -> (153.5312, 175.2631) centre (185.8847, 127.137) ccw projected
  arc A419 (153.5312, 175.2631) -> (151.2044, 177.2744) centre (0, 0) ccw projected
  arc A420 (151.2044, 177.2744) -> (154.6009, 186.1788) centre (98.9035, 202.3241) ccw projected
  arc A421 (154.6009, 186.1788) -> (152.13, 188.2033) centre (0, 0) ccw projected
  arc A422 (152.13, 188.2033) -> (144.0677, 183.1216) centre (178.916, 136.77) ccw projected
  arc A423 (144.0677, 183.1216) -> (141.638, 185.0072) centre (0, 0) ccw projected
  arc A424 (141.638, 185.0072) -> (144.5598, 194.0785) centre (88.088, 207.2618) ccw projected
  arc A425 (144.5598, 194.0785) -> (141.9855, 195.9697) centre (0, 0) ccw projected
  arc A426 (141.9855, 195.9697) -> (134.2026, 190.4696) centre (171.4485, 146.0217) ccw projected
  arc A427 (134.2026, 190.4696) -> (131.6768, 192.2244) centre (0, 0) ccw projected
  arc A428 (131.6768, 192.2244) -> (134.1158, 201.4372) centre (77.0269, 211.6218) ccw projected
  arc A429 (134.1158, 201.4372) -> (131.4452, 203.1899) centre (0, 0) ccw projected
  arc A430 (131.4452, 203.1899) -> (123.9635, 197.2867) centre (163.5033, 154.8665) ccw projected
  arc A431 (123.9635, 197.2867) -> (121.3486, 198.9058) centre (0, 0) ccw projected
  arc A432 (121.3486, 198.9058) -> (123.298, 208.2345) centre (65.7511, 215.3921) ccw projected
  arc A433 (123.298, 208.2345) -> (120.5386, 209.8438) centre (0, 0) ccw projected
  arc A434 (120.5386, 209.8438) -> (113.3788, 203.554) centre (155.1023, 163.2796) ccw projected
  arc A435 (113.3788, 203.554) -> (110.6821, 205.0328) centre (0, 0) ccw projected
  arc A436 (110.6821, 205.0328) -> (112.1365, 214.4514) centre (54.2921, 218.5619) ccw projected
  arc A437 (112.1365, 214.4514) -> (109.2961, 215.9129) centre (0, 0) ccw projected
  arc A438 (109.2961, 215.9129) -> (102.4782, 209.254) centre (146.269, 171.2376) ccw projected
  arc A439 (102.4782, 209.254) -> (99.7072, 210.5884) centre (0, 0) ccw projected
  arc A440 (99.7072, 210.5884) -> (100.6625, 220.0706) centre (42.6818, 221.1226) ccw projected
  arc A441 (100.6625, 220.0706) -> (97.7489, 221.3801) centre (0, 0) ccw projected
  arc A442 (97.7489, 221.3801) -> (91.2919, 214.3707) centre (137.028, 178.7184) ccw projected
  arc A443 (91.2919, 214.3707) -> (88.4544, 215.557) centre (0, 0) ccw projected
  arc A444 (88.4544, 215.557) -> (88.9079, 225.0764) centre (30.9525, 223.067) ccw projected
  arc A445 (88.9079, 225.0764) -> (85.9292, 226.2303) centre (0, 0) ccw projected
  arc A446 (85.9292, 226.2303) -> (79.8512, 218.8899) centre (127.4051, 185.701) ccw projected
  arc A447 (79.8512, 218.8899) -> (76.955, 219.9248) centre (0, 0) ccw projected
  arc A448 (76.955, 219.9248) -> (76.9055, 229.4549) centre (19.1369, 224.3897) ccw projected
  arc A449 (76.9055, 229.4549) -> (73.8701, 230.45) centre (0, 0) ccw projected
  arc A450 (73.8701, 230.45) -> (68.188, 222.799) centre (117.4271, 192.1661) ccw projected
  arc A451 (68.188, 222.799) -> (65.2412, 223.6797) centre (0, 0) ccw projected
  arc A452 (65.2412, 223.6797) -> (64.6888, 233.1938) centre (7.268, 225.0869) ccw projected
  arc A453 (64.6888, 233.1938) -> (61.6051, 234.0274) centre (0, 0) ccw projected
  arc A454 (61.6051, 234.0274) -> (56.3346, 226.0872) centre (107.1219, 198.0956) ccw projected
  arc A455 (56.3346, 226.0872) -> (53.3455, 226.8111) centre (0, 0) ccw projected
  arc A456 (53.3455, 226.8111) -> (52.2918, 236.2828) centre (-4.6212, 225.1568) ccw projected
  arc A457 (52.2918, 236.2828) -> (49.1684, 236.9525) centre (0, 0) ccw projected
  arc A458 (49.1684, 236.9525) -> (44.3243, 228.7452) centre (96.518, 203.4729) ccw projected
  arc A459 (44.3243, 228.7452) -> (41.3011, 229.3103) centre (0, 0) ccw projected
  arc A460 (41.3011, 229.3103) -> (39.749, 238.7133) centre (-16.4975, 224.5992) ccw projected
  arc A461 (39.749, 238.7133) -> (36.5946, 239.2171) centre (0, 0) ccw projected
  arc A462 (36.5946, 239.2171) -> (32.1904, 230.7656) centre (85.6452, 208.2831) ccw projected
  arc A463 (32.1904, 230.7656) -> (29.1416, 231.1704) centre (0, 0) ccw projected
  arc A464 (29.1416, 231.1704) -> (27.0954, 240.4784) centre (-28.3278, 223.4155) ccw projected
  arc A465 (27.0954, 240.4784) -> (23.9188, 240.8151) centre (0, 0) ccw projected
  arc A466 (23.9188, 240.8151) -> (19.9668, 232.1429) centre (74.5336, 212.5128) ccw projected
  arc A467 (19.9668, 232.1429) -> (16.9009, 232.3862) centre (0, 0) ccw projected
  arc A468 (16.9009, 232.3862) -> (14.3663, 241.5732) centre (-40.0791, 221.6091) ccw projected
  arc A469 (14.3663, 241.5732) -> (11.1764, 241.7418) centre (0, 0) ccw projected
  arc A470 (11.1764, 241.7418) -> (7.6876, 232.8731) centre (63.2143, 216.1502) ccw projected
  arc A471 (7.6876, 232.8731) -> (4.6131, 232.9543) centre (0, 0) ccw projected
  arc A472 (4.6131, 232.9543) -> (1.5972, 241.9947) centre (-51.7188, 219.1851) ccw projected
  arc A473 (1.5972, 241.9947) -> (-1.5972, 241.9947) centre (0, 0) ccw projected
  arc A474 (-1.5972, 241.9947) -> (-4.6131, 232.9543) centre (51.7188, 219.1851) ccw projected
  arc A475 (-4.6131, 232.9543) -> (-7.6876, 232.8731) centre (0, 0) ccw projected
  arc A476 (-7.6876, 232.8731) -> (-11.1764, 241.7418) centre (-63.2143, 216.1502) ccw projected
  arc A477 (-11.1764, 241.7418) -> (-14.3663, 241.5732) centre (0, 0) ccw projected
  line L5 (-10, 31.1421) -> (10, 31.1421)
  line L6 (-10, 43.1421) -> (-10, 31.1421)
  line L7 (10, 43.1421) -> (-10, 43.1421)
  line L8 (10, 31.1421) -> (10, 43.1421)
  point P0 (36.1421, -10)
  point P1 (36.1421, 10)
  point P2 (10, 36.1421)
  point P3 (10, 36.1421)
  point P4 (-10, 36.1421)
  dimension "d49" = 75
  dimension "d50" = 120
  dimension "d53" = 20
  dimension "d54" = 12
  dimension "d55" = 5
  dimension "d91" = 90
  constraints: 16 end point, 2 coincident, 2 parallel, 2 point on line, 1 centre point, 1 horizontal, 1 perpendicular, 14 other
  measures "d50" diameter of A1
  measures "d53" distance of L2.end L0.start
  measures "d54" distance of L1.end L2.end
  measures "d55" distance of L1.end point (36.142, -10)
extrude "拉伸2" add sketch "草图3" along normal blind 8.5 and the other way blind 81.5 contours A0 L2 L1 L0 | A0 L0 L3 L2 | L0 L1 L2 A0 L6 L5 L8 | L8 L5 L6 A0 | A0 L6 L7 L8 | A1
extrude "拉伸9" cut sketch "草图3" along normal through all both and the other way through all contours A0 L2 L1 L0 | L0 L1 L2 A0 L6 L5 L8 | L8 L5 L6 A0 | A0 L6 L7 L8
ref_plane "工作平面11" through (0, 59, 0) normal (0, 1, 0) x (-1, 0, 0)
sketch "草图5" plane through (0, 59, 0) normal (0, 1, 0) x (-1, 0, 0)
  line L0 (5, 10) -> (-5, 10)
  line L1 (-5, 10) -> (-5, 63)
  line L2 (-5, 63) -> (5, 63)
  line L3 (5, 63) -> (5, 10)
  line L4 (-30, 30.5) -> (30, 30.5)
  line L5 (30, 30.5) -> (30, 42.5)
  line L6 (30, 42.5) -> (-30, 42.5)
  line L7 (-30, 42.5) -> (-30, 30.5)
  line L8 (0, -26.5) -> (0, 99.5) construction
  line L9 (340.8047, 0) -> (-350.8651, 0) construction
  line L10 (10.9087, 73) -> (234.6977, 73) construction
  line L11 (-234.6977, 73) -> (-10.9087, 73) construction
  line L12 (-234.6977, 0) -> (-234.6977, 73) projected
  line L13 (-10.9087, 0) -> (-234.6977, 0) construction
  line L14 (-10.9087, 73) -> (-10.9087, 81.5) construction
  line L15 (234.6977, 73) -> (234.6977, 0) projected
  line L16 (234.6977, 0) -> (10.9087, 0) construction
  line L17 (234.6977, 36.5) -> (-252.0551, 36.5) construction
  line L18 (-10.9087, 81.5) -> (10.9087, 81.5) projected
  line L19 (10.9087, 81.5) -> (10.9087, 73) projected
  line L20 (10.9087, -8.5) -> (-10.9087, -8.5) projected
  line L21 (10.9087, 0) -> (10.9087, -8.5) projected
  line L22 (-10.9087, -8.5) -> (-10.9087, 0) projected
  point P0 (0, 0)
  dimension "d69" = 10
  dimension "d70" = 53
  dimension "d71" = 12
  dimension "d72" = 60
  constraints: 18 end point, 6 parallel, 3 horizontal, 2 perpendicular, 1 midpoint, 5 other
  measures "d69" distance of L0.start L0.end
  measures "d70" distance of L0.end L1.end
  measures "d71" distance of L6.end L4.start
  measures "d72" distance of L4.start L4.end
sketch "草图6" plane through (0, 0, 0) normal (0, 0, -1) x (-1, 0, 0)
  circle A0 centre (0, 0) radius 238
  arc A1 (-36.1421, -10) -> (-36.1421, 10) centre (0, 0) ccw projected
  circle A2 centre (0, 0) radius 226
  circle A3 centre (0, 0) radius 60
  dimension "d73" = 476
  dimension "d74" = 452
  constraints: 3 centre point, 3 coincident
  measures "d73" diameter of A0
  measures "d74" diameter of A2
extrude "拉伸4" cut sketch "草图6" against normal through all contours A2
ref_plane "工作平面12" through (0, 227, 0) normal (0, 1, 0) x (-1, 0, 0)